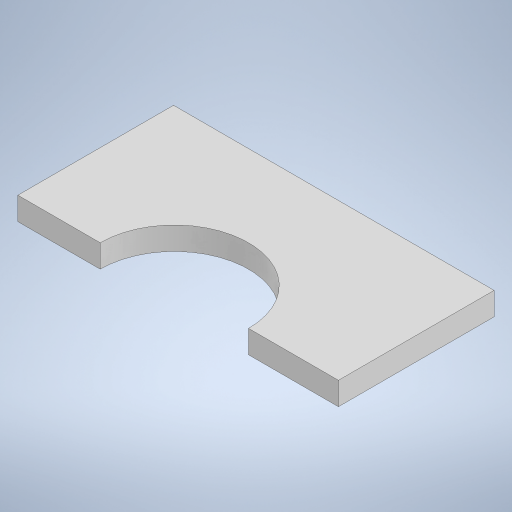
# Autodesk Inventor part: InventorPart1Commit2
Saved by Autodesk Inventor 2023 (Build 270158000, 158)
## iProperties
Created: 2023-03-15
Part Number: InventorPart1Commit2
Material: Generic
Document SubType Name: Modeling
Designer: ianjo
Density: 1 g/cm^3
Appearance: Default
Author: ianjo
Autodesk Inventor part; units mm, degrees
ref_plane "YZ Plane" through (0, 0, 0) normal (1, 0, 0) x (0, 1, 0)
ref_plane "XZ Plane" through (0, 0, 0) normal (0, 1, 0) x (-1, 0, 0)
ref_plane "XY Plane" through (0, 0, 0) normal (0, 0, 1) x (1, 0, 0)
sketch "Sketch1" plane through (0, 0, 0) normal (0, 1, 0) x (-1, 0, 0)
  line L0 (43.4289, -18.5999) -> (-45.4711, -18.5999)
  line L1 (-45.4711, -18.5999) -> (-45.4711, 24.5801)
  line L2 (-45.4711, 24.5801) -> (43.4289, 24.5801)
  line L3 (43.4289, 24.5801) -> (43.4289, -18.5999)
  point P0 (0, 0)
  dimension "d2" = 88.9
  dimension "d3" = 43.18
  constraints: 8 end point, 2 parallel, 1 horizontal, 1 perpendicular
  measures "d2" distance of L1.end L2.end
  measures "d3" distance of L0.end L1.end
extrude "Extrusion1" add sketch "Sketch1" along normal blind 6.35
sketch "Sketch2" plane through (0, 6.35, 0) normal (0, 1, 0) x (1, 0, 0)
  point P0 (0, 0)
  point P1 (-0.0268, -24.5835)
hole "Hole1" at (-0.0268, 6.35, 24.5835) direction (0, -1, 0) diameter 41.148 end through all
body "Solid1"
